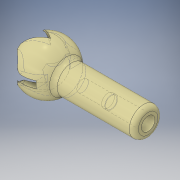
# Autodesk Inventor part: Ball
Saved by Autodesk Inventor 2016 (Build 200138000, 138)
## iProperties
Created: 2016-10-13
Part Number: Ball
Material: Generic
Document SubType Name: Modeling
Designer: desirw
Density: 1 g/cm^3
Appearance: Default
Author: desirw
Autodesk Inventor part; units mm, degrees
ref_plane "YZ Plane" through (0, 0, 0) normal (1, 0, 0) x (0, 1, 0)
ref_plane "XZ Plane" through (0, 0, 0) normal (0, 1, 0) x (-1, 0, 0)
ref_plane "Work Plane1" through (8.7249, 0, 0) normal (1, 0, 0) x (0, 1, 0)
sketch "Sketch2" plane through (8.7249, 0, 0) normal (1, 0, 0) x (0, 1, 0)
  circle A0 centre (0, 0) radius 6.35
  dimension "d21" = 12.7
  constraints: 1 centre point, 1 coincident
  measures "d21" diameter of A0
extrude "OUter Shell" add sketch "Sketch2" along normal blind 44.6278
sketch "Sketch3" plane through (8.7249, 0, 0) normal (-1, 0, 0) x (0, 0, 1)
  arc A0 (11.176, 0) -> (-11.176, 0) centre (0, 0) ccw
  line L0 (-11.176, 0) -> (11.176, 0)
  dimension "d57" = 22.352
  constraints: 2 end point, 2 point on circle, 1 centre point, 1 coincident, 1 horizontal
  measures "d57" distance of L0.start L0.end
revolve "Revolution2" add sketch "Sketch3" angle 360 about axis through (8.7249, 0, -11.176) along (0, 0, 1)
ref_plane "Work Plane8" through (5.5499, 0, 0) normal (1, 0, 0) x (0, 1, 0)
sketch "Sketch5" plane through (5.5499, 0, 0) normal (1, 0, 0) x (0, 1, 0)
  arc A0 (0, 9.5631) -> (0, -9.5631) centre (0, 0) ccw
  line L0 (0, 9.5631) -> (0, -9.5631)
  dimension "d12" = 19.1262
  constraints: 2 end point, 2 point on circle, 1 centre point, 1 coincident, 1 vertical
  measures "d12" diameter of A0
revolve "Inner Shell" cut sketch "Sketch5" angle 360 about axis through (5.5499, 0, 9.5631) along (0, 0, -1)
ref_plane "Work Plane9" through (0, 0, 11.1125) normal (0, 0, 1) x (1, 0, 0)
sketch "Sketch7" plane through (0, 0, 11.1125) normal (0, 0, 1) x (1, 0, 0)
  ellipse E0 centre (3.175, 0) end of major axis (3.175, 5.4125) minor radius 3.3411
  point P0 (0, 0)
  constraints: 2 other
extrude "Oval Expansion" cut sketch "Sketch7" against normal blind 25.4
sketch "Sketch8" plane through (53.3527, 0, 0) normal (1, 0, 0) x (0, 0, -1)
  circle A0 centre (0, 0) radius 2.9972
  dimension "d20" = 5.9944
  constraints: 1 centre point, 1 coincident
  measures "d20" diameter of A0
ref_plane "Work Plane15" through (39.3954, 0, 0) normal (1, 0, 0) x (0, 1, 0)
sketch "Sketch10" plane through (39.3954, 0, 0) normal (1, 0, 0) x (0, 1, 0)
  circle A0 centre (0, 0) radius 2.8702
  dimension "d29" = 5.7404
  constraints: 1 centre point, 1 coincident
  measures "d29" diameter of A0
extrude "Extrusion4" cut sketch "Sketch10" against normal blind 3.81
sketch "Sketch12" plane through (0, 0, 0) normal (0, 0, 1) x (1, 0, 0)
  line L0 (6.096, 1.524) -> (13.716, 1.524)
  line L1 (13.716, 1.524) -> (13.716, -1.524)
  line L2 (13.716, -1.524) -> (6.096, -1.524)
  line L3 (6.096, -1.524) -> (6.096, 1.524)
  point P0 (0, 0)
  dimension "d39" = 7.62
  constraints: 8 end point, 2 parallel, 1 horizontal, 1 perpendicular
  measures "d39" distance of L1.end L2.end
extrude "Extrusion6" cut sketch "Sketch12" along normal through all both and the other way through all
ref_plane "Work Plane12" through (37.0332, 0, 0) normal (1, 0, 0) x (0, 1, 0)
sketch "Sketch13" plane through (37.0332, 0, 0) normal (1, 0, 0) x (0, 1, 0)
  circle A0 centre (0, 0) radius 2.8702
  dimension "d41" = 5.7404
  constraints: 1 centre point, 1 coincident
  measures "d41" diameter of A0
loft "Loft2" cut profiles "Sketch8" section 2 edges at (35.5854, -2.8702, 0)
sketch "Sketch14" plane through (37.0332, 0, 0) normal (1, 0, 0) x (0, 1, 0)
  circle A0 centre (0, 0) radius 2.54
  dimension "d46" = 5.08
  constraints: 1 centre point, 1 coincident
  measures "d46" diameter of A0
extrude "Extrusion7" add sketch "Sketch13" against normal blind 12.7
extrude "Extrusion8" cut sketch "Sketch14" against normal blind 12.7
sketch "Sketch17" plane through (0, 0, 11.1125) normal (0, 0, 1) x (1, 0, 0)
  line L0 (1.8697, 4.9823) -> (1.8697, 8.8266) projected
  line L1 (17.9217, -6.35) -> (17.9217, 6.35) projected
  line L2 (1.8697, 14.5577) -> (17.8451, 14.5577)
  line L3 (9.8574, 14.5577) -> (9.8574, -13.0631)
  line L4 (1.8697, -8.8266) -> (1.8697, -4.9823) projected
  line L5 (1.8697, 8.8266) -> (9.8574, 0.059)
  line L6 (9.8574, 0.059) -> (1.8697, -8.8266)
  point P0 (0, 0)
  dimension "d60" = 16.052
  constraints: 8 end point, 1 coincident, 1 horizontal, 1 midpoint, 1 point on line, 1 vertical
  measures "d60" distance between parallel lines of L0 L1
sketch "Sketch18" plane through (0, 0, 0) normal (0, 0, 1) x (1, 0, 0)
  line L0 (1.8697, 4.9823) -> (1.8697, 8.8266) projected
  line L1 (5.5499, 0) -> (1.8697, 8.8266)
  line L2 (1.8697, 8.8266) -> (1.8697, -8.8266)
  arc A0 (1.8697, -8.8266) -> (1.8697, 8.8266) centre (5.5499, 0) ccw projected
  line L3 (1.8697, -8.8266) -> (1.8697, -4.9823) projected
  line L4 (5.5499, 0) -> (1.8697, -8.8266)
  point P0 (0, 0)
  constraints: 6 end point, 1 collinear, 1 point on circle
sketch "Sketch19" plane through (0, 0, 0) normal (0, 1, 0) x (-1, 0, 0)
  line L0 (-10.1859, 0) -> (-2.5311, 0) construction
  line L1 (-10.1859, 0) -> (-3.9661, 0) construction
  line L2 (-10.1859, 0) -> (-3.0039, 0) construction
  line L3 (-10.1859, 0) -> (-0.3588, 5.6737)
  line L4 (-10.1859, 0) -> (1.1615, 0) construction
  line L5 (-0.3588, 5.6737) -> (-0.3588, -5.6737)
  line L6 (-10.1859, 0) -> (-0.3588, -5.6737)
  line L7 (-10.1859, 0) -> (0.1303, 0) construction
  point P0 (0, 0)
  dimension "d65" = 30
  dimension "d66" = 30
  constraints: 16 end point, 5 horizontal, 1 equal length, 1 vertical
  measures "d65" angle of L4 L3
  measures "d66" angle of L6 L7
extrude "Extrusion10" cut sketch "Sketch19" along normal mid plane 25.4
pattern_circular "Circular Pattern1" count 4 over 360 about axis through (8.7249, 0, 0) along (1, 0, 0) of "Extrusion10"
fillet "Fillet1" radius 3.175 1 edges at (17.9217, -6.35, 0)
fillet "Fillet2" radius 2.032 1 edges at (53.3527, -6.35, 0)
chamfer "Chamfer1" distance 1.27 angle 45 8 edges at (5.1129, 4.409, 8.4748) (2.5053, 5.3026, 7.3529) (4.0297, -5.2324, 7.859) (5.9079, -3.1137, 9.0349) (4.0297, -5.2324, -7.859) (5.9079, -3.1137, -9.0349) (2.5053, 5.3026, -7.3529) (5.1129, 4.409, -8.4748)
body "Solid1"
